antennatripod (Autodesk Fusion 360 design; units mm, degrees)
Autodesk Fusion 360 part; units mm, degrees
sketch "Sketch1" plane through (0, 0, 0) normal (0, 0, 1) x (1, 0, 0)
  line L0 (0, 0) -> (0, 51.9615)
  line L1 (-30, 51.9615) -> (30, 51.9615)
  line L2 (60, 0) -> (30, -51.9615)
  line L3 (-30, -51.9615) -> (-60, 0)
  arc A0 (60, 0) -> (30, 51.9615) centre (0, 0) ccw
  arc A1 (-30, 51.9615) -> (-60, 0) centre (0, 0) ccw
  arc A2 (-30, -51.9615) -> (30, -51.9615) centre (0, 0) ccw
  circle A3 centre (0, 0) radius 6.5
  line L4 (0, 0) -> (34.641, 20)
  line L5 (34.641, 20, 0) -> (49.225, 28.4201, 4.3095)
  circle A4 through (51.0012, 22.171, 3.7321) (32.6711, 33.4119, 0) (33.241, 11.9171, -3.7321)
  line L6 (38.9711, 22.5) -> (27.3672, -2.6014)
  circle A5 through (54.4861, 22.0756, 4.8132) (30.8461, 36.5729, 0) (31.5811, 8.8514, -4.8132)
  circle A6 through (-26.941, 22.829, -3.7321) (-44.7012, 33.0829, 3.7321) (-45.2711, 11.5881, 0)
  line L7 (-19.399, 11.2) -> (-11.4307, 25.0014)
  circle A7 through (-23.4561, 22.9244, -4.8132) (-46.3611, 36.1486, 4.8132) (-47.0961, 8.4271, 0)
  circle A8 through (12.6, -45, 0) (-6.3, -34.7461, -3.7321) (-6.3, -55.2539, 3.7321)
  line L8 (0, -22.4) -> (-15.9365, -22.4)
  circle A9 through (16.25, -45, 0) (-8.125, -31.7758, -4.8132) (-8.125, -58.2242, 4.8132)
  line L9 (34.641, 20) -> (51.9615, 30)
  line L10 (51.9615, 30) -> (38.9711, 22.5)
  line L11 (0, 0) -> (-51.9615, 30)
  line L12 (0, 0) -> (0, -60)
  line L13 (-51.9615, 30) -> (-38.9711, 22.5)
  line L14 (0, -60) -> (0, -45)
  line L15 (0, 0) -> (45, -25.9808)
  line L16 (0, 0) -> (0, 51.9615)
  line L17 (0, 0) -> (-45, -25.9808)
  circle A10 centre (39.4445, -22.7733) radius 3
  circle A11 centre (0, 45.5466) radius 3
  circle A12 centre (-39.4445, -22.7733) radius 3
  circle A13 centre (28.2256, -35.1273) radius 3
  dimension "d4" = 13
  dimension "d10" = 25.2
  dimension "d34" = 15
  dimension "d35" = 15
  dimension "d36" = 15
  dimension "d40" = 360
  dimension "d41" = 6
  dimension "d43" = 360
  dimension "d44" = 6
  dimension "d47" = 32.5
  dimension "d48" = 32.5
  dimension "d49" = 32.5
  constraint coincident L0.start A0.centre
  constraint coincident L1 L0.end
  constraint concentric A0 A1
  constraint concentric A1 A2
  constraint coincident L6.start L10.end
  constraint midpoint A0 L9.end
  constraint parallel L4 L9
  constraint parallel L9 L10
  constraint midpoint A1 L11.end
  constraint midpoint A2 L12.end
  constraint parallel L0 L12
  constraint parallel L11 L13
  constraint parallel L12 L14
  constraint midpoint L2 L15.end
  constraint perpendicular L2 L15
  constraint coincident L15 A10.centre
  measures "d4" diameter of A3
  measures "d34" distance of L9.end L6.start
  measures "d35" distance of L11.end L13.end
  measures "d36" distance of L12.end L14.end
  measures "d41" diameter of A10
  measures "d44" diameter of A13
extrude "Extrude1" add sketch "Sketch1" along normal blind 8 contours L0 L1 A1 A3 L11 L13 L16 A11 | L0 L1 A0 A3 L4 L9 L10 L16 A11 | L2 A0 A3 L4 L9 L10 L15 A10 | L3 A1 A3 L11 L13 L17 A12 | L3 A2 A3 L12 L14 L17 A12 | L2 A2 A3 L12 L14 L15 A10 | L0 L16 A11 | L0 L16 A11 | L15 A10 | L15 A10 | L17 A12 | L17 A12 | A13
extrude "Extrude2" cut sketch "Sketch1" against normal blind 50 contours A5 in plane through (4.5588, 2.632, -14.4627) normal (-0.296198, -0.17101, 0.939693)
extrude "Extrude3" add sketch "Sketch1" against normal blind 50 contours A5 in plane through (4.5588, 2.632, -14.4627) normal (-0.296198, -0.17101, 0.939693)
extrude "Extrude4" cut sketch "Sketch1" against normal blind 50 contours A9 in plane through (0, -5.264, -14.4627) normal (0, 0.34202, 0.939693)
extrude "Extrude5" add sketch "Sketch1" against normal blind 50 contours A9 in plane through (0, -5.264, -14.4627) normal (0, 0.34202, 0.939693)
extrude "Extrude6" cut sketch "Sketch1" against normal blind 50 contours A7 in plane through (-4.5588, 2.632, -14.4627) normal (0.296198, -0.17101, 0.939693)
extrude "Extrude7" add sketch "Sketch1" against normal blind 50 contours A7 in plane through (-4.5588, 2.632, -14.4627) normal (0.296198, -0.17101, 0.939693)
extrude "Extrude8" add sketch "Sketch1" along normal blind 5 contours A7 in plane through (-4.5588, 2.632, -14.4627) normal (0.296198, -0.17101, 0.939693)
extrude "Extrude9" add sketch "Sketch1" along normal blind 5 contours A5 in plane through (4.5588, 2.632, -14.4627) normal (-0.296198, -0.17101, 0.939693)
extrude "Extrude10" add sketch "Sketch1" along normal blind 6 contours A9 in plane through (0, -5.264, -14.4627) normal (0, 0.34202, 0.939693)
sketch "Sketch5" plane through (0, 0, 0) normal (0, 1, 0) x (1, 0, 0)
  line L0 (30, 0) -> (-30, 0)
  line L1 (-30, 0) -> (-30, -8)
  line L2 (-30, -8) -> (30, -8)
  line L3 (30, -8) -> (30, 0)
  line L4 (-30, -8) -> (-59.8416, -8)
  line L5 (30, -8) -> (35.4636, -8)
  line L6 (59.9189, -29.3095) -> (-59.8416, -29.3095)
  line L7 (-59.8416, -29.3095) -> (-59.8416, -8)
  line L8 (-59.8416, -8) -> (59.9189, -8)
  line L9 (59.9189, -8) -> (59.9189, -29.3095)
  constraint coincident L1.end L2.start
  constraint perpendicular L1 L4
  constraint coincident L2.end L3.start
  constraint perpendicular L3 L5
  constraint horizontal L6
  constraint vertical L7
  constraint horizontal L8
  constraint vertical L9
extrude "Extrude11" cut sketch "Sketch5" along normal mid plane 80 contours L2 L4 L5 L6 L7 L8 L9
extrude "Extrude12" cut sketch "Sketch5" along normal mid plane 126 contours L2 L4 L5 L6 L7 L8 L9
extrude "Extrude13" cut sketch "Sketch1" along normal blind 15 contours L0 L16 A11 | L0 L16 A11 | L15 A10 | L15 A10 | L17 A12 | L17 A12 | A13
